Autodesk Inventor part; units mm, degrees
(part 4 of 5)
sketch "Эскиз10" plane through (0, 2, 0) normal (0, 1, 0) x (1, 0, 0)
  circle A0 centre (0, -54) radius 1.6 construction
  line L0 (0, -54) -> (0, -66.038) construction
  line L1 (-10.11, -19.198) -> (10.11, -19.198) construction
  line L2 (10.11, -19.198) -> (10.11, -35.5658) construction
  line L3 (10.11, -58.698) -> (-10.11, -58.698) construction
  line L4 (-10.11, -58.698) -> (-10.11, -55.0209) construction
  circle A1 centre (31.9203, -33.1335) radius 1.6 construction
  circle A2 centre (-31.9203, -33.1335) radius 1.6 construction
  circle A3 centre (21.9203, -33.1335) radius 1.6 construction
  circle A4 centre (-21.9203, -33.1335) radius 1.6 construction
  line L5 (16.2132, -33.1838) -> (7.7166, -24.6871) construction
  arc A5 (8.4003, -21.4111) -> (7.7166, -24.6871) centre (9.1308, -23.2729) ccw construction
  arc A6 (8.4003, -21.4111) -> (21.4111, -8.4003) centre (0, 0) ccw construction
  arc A7 (24.6871, -7.7166) -> (21.4111, -8.4003) centre (23.2729, -9.1308) ccw construction
  line L6 (24.6871, -7.7166) -> (37.8302, -20.8597) construction
  arc A8 (37.8302, -23.6881) -> (37.8302, -20.8597) centre (36.416, -22.2739) ccw construction
  line L7 (37.8302, -23.6881) -> (33.2132, -28.3051) construction
  line L8 (33.2132, -28.3051) -> (21.9203, -28.3051) construction
  arc A9 (21.9203, -28.3051) -> (20.5061, -28.8909) centre (21.9203, -30.3051) ccw construction
  line L9 (20.5061, -28.8909) -> (16.2132, -33.1838) construction
  line L10 (-31.4801, -37.1092) -> (-27.2236, -41.3657) construction
  arc A10 (-27.2236, -44.1942) -> (-27.2236, -41.3657) centre (-28.6378, -42.78) ccw construction
  line L11 (-27.2236, -44.1942) -> (-46.669, -63.6396) construction
  line L12 (-46.669, -63.6396) -> (-63.6396, -46.669) construction
  line L13 (-63.6396, -46.669) -> (-44.1942, -27.2236) construction
  arc A11 (-41.3657, -27.2236) -> (-44.1942, -27.2236) centre (-42.78, -28.6378) ccw construction
  line L14 (-41.3657, -27.2236) -> (-35.896, -32.6933) construction
  arc A12 (-35.896, -32.6933) -> (-31.4801, -37.1092) centre (-31.9203, -33.1335) ccw construction
  circle A13 centre (45.1111, -90.3659) radius 1.6 construction
  circle A14 centre (-45.1111, 90.3659) radius 1.6 construction
  circle A15 centre (-90.3659, 45.1111) radius 1.6 construction
  circle A16 centre (90.3659, -45.1111) radius 1.6 construction
  circle A17 centre (-45.1111, -90.3659) radius 1.6 construction
  circle A18 centre (45.1111, 90.3659) radius 1.6 construction
  circle A19 centre (-90.3659, -45.1111) radius 1.6 construction
  circle A20 centre (90.3659, 45.1111) radius 1.6 construction
  circle A21 centre (101, 0) radius 1.6 construction
  circle A22 centre (-101, 0) radius 1.6 construction
  arc A23 (90.4395, -37.7453) -> (97.9653, -2.6059) centre (0, 0) ccw construction
  arc A24 (87.1795, -38.3892) -> (90.4395, -37.7453) centre (88.5938, -36.975) ccw construction
  line L15 (87.1795, -38.3892) -> (83.085, -34.2947) construction
  arc A25 (83.085, -34.2947) -> (76.014, -34.2947) centre (79.5495, -37.8302) ccw construction
  line L16 (76.014, -34.2947) -> (67.8823, -42.4264) construction
  line L17 (67.8823, -42.4264) -> (47.1257, -21.6698) construction
  arc A26 (47.1257, -21.6698) -> (43.384, -17.9282) centre (43.1335, -21.9203) ccw construction
  line L18 (43.384, -17.9282) -> (26.8701, -1.4142) construction
  arc A27 (26.8701, 1.4142) -> (26.8701, -1.4142) centre (28.2843, 0) ccw construction
  line L19 (26.8701, 1.4142) -> (43.384, 17.9282) construction
  arc A28 (43.384, 17.9282) -> (47.1257, 21.6698) centre (43.1335, 21.9203) ccw construction
  line L20 (47.1257, 21.6698) -> (67.8823, 42.4264) construction
  line L21 (67.8823, 42.4264) -> (76.014, 34.2947) construction
  arc A29 (76.014, 34.2947) -> (83.085, 34.2947) centre (79.5495, 37.8302) ccw construction
  line L22 (83.085, 34.2947) -> (87.1795, 38.3892) construction
  arc A30 (90.4395, 37.7453) -> (87.1795, 38.3892) centre (88.5938, 36.975) ccw construction
  arc A31 (97.9653, 2.6059) -> (90.4395, 37.7453) centre (0, 0) ccw construction
  arc A32 (97.9653, 2.6059) -> (97.9653, -2.6059) centre (101, 0) ccw construction
  arc A33 (3.4868, -52.0398) -> (5.1776, -53.4237) centre (6.1018, -50.5696) ccw projected
  arc A34 (3.4868, -52.0398) -> (-3.4868, -52.0398) centre (0, -54) ccw projected
  arc A35 (-5.1776, -53.4237) -> (-3.4868, -52.0398) centre (-6.1018, -50.5696) ccw projected
  line L23 (-5.1776, -53.4237) -> (-14.5119, -56.4463) projected
  arc A36 (-15.1585, -56.5907) -> (-14.5119, -56.4463) centre (-15.6055, -53.069) ccw projected
  line L24 (-15.1585, -56.5907) -> (-20.596, -57.2809) construction
  line L25 (-20.596, -57.2809) -> (-26.2105, -51.6664) projected
  line L26 (-26.2105, -51.6664) -> (-21.6698, -47.1257) projected
  arc A37 (-21.6698, -47.1257) -> (-17.9282, -43.384) centre (-21.9203, -43.1335) ccw projected
  line L27 (-17.9282, -43.384) -> (-1.4142, -26.8701) projected
  arc A38 (1.4142, -26.8701) -> (-1.4142, -26.8701) centre (0, -28.2843) ccw projected
  line L28 (1.4142, -26.8701) -> (17.9282, -43.384) projected
  arc A39 (17.9282, -43.384) -> (21.6698, -47.1257) centre (21.9203, -43.1335) ccw projected
  line L29 (21.6698, -47.1257) -> (26.2105, -51.6664) projected
  line L30 (26.2105, -51.6664) -> (20.596, -57.2809) projected
  line L31 (20.596, -57.2809) -> (15.1585, -56.5907) projected
  arc A40 (14.5119, -56.4463) -> (15.1585, -56.5907) centre (15.6055, -53.069) ccw construction
  line L32 (14.5119, -56.4463) -> (5.1776, -53.4237) projected
  line L33 (63.6396, 46.669) -> (44.1942, 27.2236) construction
  arc A41 (41.3657, 27.2236) -> (44.1942, 27.2236) centre (42.78, 28.6378) ccw construction
  line L34 (41.3657, 27.2236) -> (27.2236, 41.3657) construction
  arc A42 (27.2236, 44.1942) -> (27.2236, 41.3657) centre (28.6378, 42.78) ccw construction
  line L35 (27.2236, 44.1942) -> (46.669, 63.6396) construction
  line L36 (46.669, 63.6396) -> (63.6396, 46.669) construction
  line L37 (-46.669, 63.6396) -> (-27.2236, 44.1942) construction
  arc A43 (-27.2236, 41.3657) -> (-27.2236, 44.1942) centre (-28.6378, 42.78) ccw construction
  line L38 (-27.2236, 41.3657) -> (-41.3657, 27.2236) construction
  arc A44 (-44.1942, 27.2236) -> (-41.3657, 27.2236) centre (-42.78, 28.6378) ccw construction
  line L39 (-44.1942, 27.2236) -> (-63.6396, 46.669) construction
  line L40 (-63.6396, 46.669) -> (-46.669, 63.6396) construction
  circle A45 centre (-21.9203, 43.1335) radius 1.6 construction
  arc A46 (-24.6871, 7.7166) -> (-21.4111, 8.4003) centre (-23.2729, 9.1308) ccw construction
  line L41 (-24.6871, 7.7166) -> (-37.8302, 20.8597) construction
  arc A47 (-37.8302, 23.6881) -> (-37.8302, 20.8597) centre (-36.416, 22.2739) ccw construction
  line L42 (-37.8302, 23.6881) -> (-23.6881, 37.8302) construction
  arc A48 (-20.8597, 37.8302) -> (-23.6881, 37.8302) centre (-22.2739, 36.416) ccw construction
  line L43 (-20.8597, 37.8302) -> (-7.7166, 24.6871) construction
  arc A49 (-8.4003, 21.4111) -> (-7.7166, 24.6871) centre (-9.1308, 23.2729) ccw construction
  arc A50 (-8.4003, 21.4111) -> (-21.4111, 8.4003) centre (0, 0) ccw construction
  line L44 (37.8302, 20.8597) -> (24.6871, 7.7166) construction
  arc A51 (21.4111, 8.4003) -> (24.6871, 7.7166) centre (23.2729, 9.1308) ccw construction
  arc A52 (21.4111, 8.4003) -> (8.4003, 21.4111) centre (0, 0) ccw construction
  arc A53 (7.7166, 24.6871) -> (8.4003, 21.4111) centre (9.1308, 23.2729) ccw construction
  line L45 (7.7166, 24.6871) -> (20.8597, 37.8302) construction
  arc A54 (23.6881, 37.8302) -> (20.8597, 37.8302) centre (22.2739, 36.416) ccw construction
  line L46 (23.6881, 37.8302) -> (37.8302, 23.6881) construction
  arc A55 (37.8302, 20.8597) -> (37.8302, 23.6881) centre (36.416, 22.2739) ccw construction
  circle A56 centre (21.9203, -43.1335) radius 1.6 construction
  circle A57 centre (-43.1335, -21.9203) radius 1.6 construction
  circle A58 centre (43.1335, 21.9203) radius 1.6 construction
  circle A59 centre (21.9203, 43.1335) radius 1.6 construction
  circle A60 centre (-21.9203, -43.1335) radius 1.6 construction
  circle A61 centre (-43.1335, 21.9203) radius 1.6 construction
  circle A62 centre (0, 0) radius 18 construction
  circle A63 centre (43.1335, -21.9203) radius 1.6 construction
  circle A64 centre (0, 22) radius 1.6 construction
  circle A65 centre (-22, 0) radius 1.6 construction
  circle A66 centre (0, -22) radius 1.6 construction
  circle A67 centre (22, 0) radius 1.6 construction
  circle A68 centre (-37.8302, 79.5495) radius 1.6 construction
  circle A69 centre (-79.5495, 37.8302) radius 1.6 construction
  circle A70 centre (-79.5495, -37.8302) radius 1.6 construction
  circle A71 centre (79.5495, -37.8302) radius 1.6 construction
  circle A72 centre (37.8302, 79.5495) radius 1.6 construction
  circle A73 centre (79.5495, 37.8302) radius 1.6 construction
  circle A74 centre (-20.5578, -60.8546) radius 1.55 construction
  circle A75 centre (20.5578, -60.8546) radius 1.55 construction
  circle A76 centre (37.8302, -79.5495) radius 1.6 construction
  circle A77 centre (-37.8302, -79.5495) radius 1.6 construction
  line L47 (-33.2132, -28.3051) -> (-37.8302, -23.6881) construction
  arc A78 (-37.8302, -20.8597) -> (-37.8302, -23.6881) centre (-36.416, -22.2739) ccw construction
  line L48 (-37.8302, -20.8597) -> (-24.6871, -7.7166) construction
  arc A79 (-21.4111, -8.4003) -> (-24.6871, -7.7166) centre (-23.2729, -9.1308) ccw construction
  arc A80 (-21.4111, -8.4003) -> (-8.4003, -21.4111) centre (0, 0) ccw projected
  arc A81 (-7.7166, -24.6871) -> (-8.4003, -21.4111) centre (-9.1308, -23.2729) ccw projected
  line L49 (-7.7166, -24.6871) -> (-16.2132, -33.1838) projected
  line L50 (-16.2132, -33.1838) -> (-20.5061, -28.8909) construction
  arc A82 (-20.5061, -28.8909) -> (-21.9203, -28.3051) centre (-21.9203, -30.3051) ccw construction
  line L51 (-21.9203, -28.3051) -> (-33.2132, -28.3051) construction
  arc A83 (37.7453, 90.4395) -> (18.0526, 96.3229) centre (0, 0) ccw construction
  arc A84 (38.3892, 87.1795) -> (37.7453, 90.4395) centre (36.975, 88.5938) ccw construction
  line L52 (38.3892, 87.1795) -> (34.2947, 83.085) construction
  arc A85 (34.2947, 83.085) -> (34.2947, 76.014) centre (37.8302, 79.5495) ccw construction
  line L53 (34.2947, 76.014) -> (42.4264, 67.8823) construction
  line L54 (42.4264, 67.8823) -> (21.6698, 47.1257) construction
  arc A86 (21.6698, 47.1257) -> (17.9282, 43.384) centre (21.9203, 43.1335) ccw construction
  line L55 (17.9282, 43.384) -> (1.4142, 26.8701) construction
  arc A87 (-1.4142, 26.8701) -> (1.4142, 26.8701) centre (0, 28.2843) ccw construction
  line L56 (-1.4142, 26.8701) -> (-17.9282, 43.384) construction
  arc A88 (-17.9282, 43.384) -> (-21.6698, 47.1257) centre (-21.9203, 43.1335) ccw construction
  line L57 (-21.6698, 47.1257) -> (-42.4264, 67.8823) construction
  line L58 (-42.4264, 67.8823) -> (-34.2947, 76.014) construction
  arc A89 (-34.2947, 76.014) -> (-34.2947, 83.085) centre (-37.8302, 79.5495) ccw construction
  line L59 (-34.2947, 83.085) -> (-38.3892, 87.1795) construction
  arc A90 (-37.7453, 90.4395) -> (-38.3892, 87.1795) centre (-36.975, 88.5938) ccw construction
  arc A91 (-18.0526, 96.3229) -> (-37.7453, 90.4395) centre (0, 0) ccw construction
  arc A92 (-14.5, 93.3742) -> (-18.0526, 96.3229) centre (-17.5, 93.3742) ccw construction
  line L60 (-14.5, 93.3742) -> (-14.5, 87) construction
  arc A93 (-14.5, 87) -> (-11.5, 84) centre (-11.5, 87) ccw construction
  line L61 (-11.5, 84) -> (11.5, 84) construction
  arc A94 (11.5, 84) -> (14.5, 87) centre (11.5, 87) ccw construction
  line L62 (14.5, 87) -> (14.5, 93.3742) construction
  arc A95 (18.0526, 96.3229) -> (14.5, 93.3742) centre (17.5, 93.3742) ccw construction
  line L63 (-24.3148, -60.6331) -> (-24.842, -61.8893) construction
  arc A96 (-25.4187, -62.8242) -> (-24.842, -61.8893) centre (-28.1154, -60.5155) ccw construction
  line L64 (-25.4187, -62.8242) -> (-34.1909, -73.0707) construction
  arc A97 (-37.1244, -73.1843) -> (-34.1909, -73.0707) centre (-35.7102, -71.7701) ccw construction
  line L65 (-37.1244, -73.1843) -> (-42.4264, -67.8823) construction
  line L66 (-42.4264, -67.8823) -> (-29.746, -55.2019) construction
  line L67 (-29.746, -55.2019) -> (-24.3148, -60.6331) construction
  line L68 (29.746, -55.2019) -> (42.4264, -67.8823) construction
  line L69 (42.4264, -67.8823) -> (37.1244, -73.1843) construction
  arc A98 (34.1909, -73.0707) -> (37.1244, -73.1843) centre (35.7102, -71.7701) ccw construction
  line L70 (34.1909, -73.0707) -> (25.4187, -62.8242) construction
  arc A99 (24.842, -61.8893) -> (25.4187, -62.8242) centre (28.1154, -60.5155) ccw construction
  line L71 (24.842, -61.8893) -> (24.3148, -60.6331) construction
  line L72 (24.3148, -60.6331) -> (29.746, -55.2019) construction
  arc A100 (-90.4395, 37.7453) -> (-97.9653, 2.6059) centre (0, 0) ccw construction
  arc A101 (-87.1795, 38.3892) -> (-90.4395, 37.7453) centre (-88.5938, 36.975) ccw construction
  line L73 (-87.1795, 38.3892) -> (-83.085, 34.2947) construction
  arc A102 (-83.085, 34.2947) -> (-76.014, 34.2947) centre (-79.5495, 37.8302) ccw construction
  line L74 (-76.014, 34.2947) -> (-67.8823, 42.4264) construction
  line L75 (-67.8823, 42.4264) -> (-47.1257, 21.6698) construction
  arc A103 (-47.1257, 21.6698) -> (-43.384, 17.9282) centre (-43.1335, 21.9203) ccw construction
  line L76 (-43.384, 17.9282) -> (-26.8701, 1.4142) construction
  arc A104 (-26.8701, -1.4142) -> (-26.8701, 1.4142) centre (-28.2843, 0) ccw construction
  line L77 (-26.8701, -1.4142) -> (-43.384, -17.9282) construction
  arc A105 (-43.384, -17.9282) -> (-47.1257, -21.6698) centre (-43.1335, -21.9203) ccw construction
  line L78 (-47.1257, -21.6698) -> (-67.8823, -42.4264) construction
  line L79 (-67.8823, -42.4264) -> (-76.014, -34.2947) construction
  arc A106 (-76.014, -34.2947) -> (-83.085, -34.2947) centre (-79.5495, -37.8302) ccw construction
  line L80 (-83.085, -34.2947) -> (-87.1795, -38.3892) construction
  arc A107 (-90.4395, -37.7453) -> (-87.1795, -38.3892) centre (-88.5938, -36.975) ccw construction
  arc A108 (-97.9653, -2.6059) -> (-90.4395, -37.7453) centre (0, 0) ccw construction
  arc A109 (-97.9653, -2.6059) -> (-97.9653, 2.6059) centre (-101, 0) ccw construction
  arc A110 (-93.0503, 48.6481) -> (-93.0503, -48.6481) centre (0, 0) ccw construction
  arc A111 (-93.0503, -48.6481) -> (-88.2704, -49.3795) centre (-90.3917, -47.2582) ccw construction
  line L81 (-88.2704, -49.3795) -> (-85.2064, -46.3155) construction
  arc A112 (-73.8927, -46.3155) -> (-85.2064, -46.3155) centre (-79.5495, -51.9723) ccw construction
  line L82 (-73.8927, -46.3155) -> (-46.3155, -73.8927) construction
  arc A113 (-46.3155, -85.2064) -> (-46.3155, -73.8927) centre (-51.9723, -79.5495) ccw construction
  line L83 (-46.3155, -85.2064) -> (-49.3795, -88.2704) construction
  arc A114 (-49.3795, -88.2704) -> (-48.6481, -93.0503) centre (-47.2582, -90.3917) ccw construction
  arc A115 (-48.6481, -93.0503) -> (-45.42, -94.668) centre (0, 0) ccw construction
  arc A116 (-45.42, -94.668) -> (-43.0355, -94.1655) centre (-44.5548, -92.8648) ccw construction
  line L84 (-43.0355, -94.1655) -> (-18.3802, -65.3664) construction
  arc A117 (-17.477, -64.7643) -> (-18.3802, -65.3664) centre (-16.8609, -66.6671) ccw construction
  line L85 (-17.477, -64.7643) -> (-0.6161, -59.3045) construction
  arc A118 (0.6161, -59.3045) -> (-0.6161, -59.3045) centre (0, -61.2072) ccw construction
  line L86 (0.6161, -59.3045) -> (17.477, -64.7643) construction
  arc A119 (18.3802, -65.3664) -> (17.477, -64.7643) centre (16.8609, -66.6671) ccw construction
  line L87 (18.3802, -65.3664) -> (43.0355, -94.1655) construction
  arc A120 (43.0355, -94.1655) -> (45.42, -94.668) centre (44.5548, -92.8648) ccw construction
  arc A121 (45.42, -94.668) -> (48.6481, -93.0503) centre (0, 0) ccw construction
  arc A122 (48.6481, -93.0503) -> (49.3795, -88.2704) centre (47.2582, -90.3917) ccw construction
  line L88 (49.3795, -88.2704) -> (46.3155, -85.2064) construction
  arc A123 (46.3155, -73.8927) -> (46.3155, -85.2064) centre (51.9723, -79.5495) ccw construction
  line L89 (46.3155, -73.8927) -> (73.8927, -46.3155) construction
  arc A124 (85.2064, -46.3155) -> (73.8927, -46.3155) centre (79.5495, -51.9723) ccw construction
  line L90 (85.2064, -46.3155) -> (88.2704, -49.3795) construction
  arc A125 (88.2704, -49.3795) -> (93.0503, -48.6481) centre (90.3917, -47.2582) ccw construction
  arc A126 (93.0503, -48.6481) -> (93.0503, 48.6481) centre (0, 0) ccw construction
  arc A127 (93.0503, 48.6481) -> (88.2704, 49.3795) centre (90.3917, 47.2582) ccw construction
  line L91 (88.2704, 49.3795) -> (85.2064, 46.3155) construction
  arc A128 (73.8927, 46.3155) -> (85.2064, 46.3155) centre (79.5495, 51.9723) ccw construction
  line L92 (73.8927, 46.3155) -> (46.3155, 73.8927) construction
  arc A129 (46.3155, 85.2064) -> (46.3155, 73.8927) centre (51.9723, 79.5495) ccw construction
  line L93 (46.3155, 85.2064) -> (49.3795, 88.2704) construction
  arc A130 (49.3795, 88.2704) -> (48.6481, 93.0503) centre (47.2582, 90.3917) ccw construction
  arc A131 (48.6481, 93.0503) -> (11.8382, 104.3305) centre (0, 0) ccw construction
  arc A132 (11.8382, 104.3305) -> (8.5, 101.3496) centre (11.5, 101.3496) ccw construction
  line L94 (8.5, 101.3496) -> (8.5, 90.5) construction
  arc A133 (7, 89) -> (8.5, 90.5) centre (7, 90.5) ccw construction
  line L95 (7, 89) -> (-7, 89) construction
  arc A134 (-8.5, 90.5) -> (-7, 89) centre (-7, 90.5) ccw construction
  line L96 (-8.5, 90.5) -> (-8.5, 101.3496) construction
  arc A135 (-8.5, 101.3496) -> (-11.8382, 104.3305) centre (-11.5, 101.3496) ccw construction
  arc A136 (-11.8382, 104.3305) -> (-48.6481, 93.0503) centre (0, 0) ccw construction
  arc A137 (-48.6481, 93.0503) -> (-49.3795, 88.2704) centre (-47.2582, 90.3917) ccw construction
  line L97 (-49.3795, 88.2704) -> (-46.3155, 85.2064) construction
  arc A138 (-46.3155, 73.8927) -> (-46.3155, 85.2064) centre (-51.9723, 79.5495) ccw construction
  line L98 (-46.3155, 73.8927) -> (-73.8927, 46.3155) construction
  arc A139 (-85.2064, 46.3155) -> (-73.8927, 46.3155) centre (-79.5495, 51.9723) ccw construction
  line L99 (-85.2064, 46.3155) -> (-88.2704, 49.3795) construction
  arc A140 (-88.2704, 49.3795) -> (-93.0503, 48.6481) centre (-90.3917, 47.2582) ccw construction
  circle A141 centre (0, -54) radius 1.6 construction
  line L100 (35.896, -32.6933) -> (41.3657, -27.2236) construction
  arc A142 (44.1942, -27.2236) -> (41.3657, -27.2236) centre (42.78, -28.6378) ccw construction
  line L101 (44.1942, -27.2236) -> (63.6396, -46.669) construction
  line L102 (63.6396, -46.669) -> (46.669, -63.6396) construction
  line L103 (46.669, -63.6396) -> (27.2236, -44.1942) construction
  arc A143 (27.2236, -41.3657) -> (27.2236, -44.1942) centre (28.6378, -42.78) ccw construction
  line L104 (27.2236, -41.3657) -> (31.4801, -37.1092) construction
  arc A144 (31.4801, -37.1092) -> (35.896, -32.6933) centre (31.9203, -33.1335) ccw construction
  line L105 (0, -22) -> (0, -54) construction
  circle A145 centre (7.01, -46.7128) radius 1.75
  circle A146 centre (-7.01, -24.698) radius 1.75
  line L106 (-16.2132, -33.1838) -> (-7.7166, -24.6871) projected
  line L107 (-11.01, -27.9806) -> (-11.01, -20.1936)
  arc A147 (-21.4111, -8.4003) -> (-8.4003, -21.4111) centre (0, 0) ccw projected
  line L108 (10.11, -35.5658) -> (10.11, -55.0209)
  line L109 (10.11, -55.0209) -> (10.11, -58.698) construction
  line L110 (-10.11, -55.0209) -> (-10.11, -35.5658)
  line L111 (-10.11, -35.5658) -> (-10.11, -19.198) construction
  line L112 (-17.9282, -43.384) -> (-17.9282, -56.9423)
  line L113 (-15.1585, -56.5907) -> (-20.596, -57.2809) projected
  line L114 (17.9282, -43.384) -> (17.9282, -56.9423)
  line L115 (-8.1, -30.338) -> (8.1, -30.338) construction
  line L116 (8.1, -30.338) -> (8.1, -60.538) construction
  line L117 (8.1, -60.538) -> (-8.1, -60.538) construction
  line L118 (-8.1, -60.538) -> (-8.1, -30.338) construction
  circle A148 centre (-3.6, -36.138) radius 1.5
  circle A149 centre (5, -40.8369) radius 1.5
  circle A150 centre (3.6, -51.4954) radius 1.5
  circle A151 centre (-5, -53.3813) radius 1.5
  point P0 (-8.553, -25.5236)
  point P1 (-7.1564, -22.9541)
  dimension "d26" = 360
  dimension "d141" = 12.038
  dimension "d142" = 7.34
  dimension "d143" = 3.5
  dimension "d145" = 39.5
  dimension "d147" = 3.5
  dimension "d148" = 3.1
  dimension "d149" = 5.5
  dimension "d150" = 26.1
  dimension "d151" = 4
  dimension "d152" = 3.1
  dimension "d153" = 20.22
  dimension "d171" = 5.5
  dimension "d172" = 30.2
  dimension "d173" = 16.2
  dimension "d174" = 3
  dimension "d175" = 4.5
  dimension "d176" = 3
  dimension "d177" = 3.1
  dimension "d178" = 5.8
  dimension "d179" = 9.8
  dimension "d180" = 3
  dimension "d181" = 4.5
  dimension "d182" = 10.75
  dimension "d183" = 3
  dimension "d184" = 3.1
  dimension "d185" = 16.0424
  dimension "d186" = 17.3
  constraints: 34 end point, 12 parallel, 6 centre point, 6 point on line, 4 perpendicular, 4 vertical, 2 horizontal, 1 point on circle, 1 symmetric about line, 2 other
  measures "d141" distance of L0.start L0.end
  measures "d142" distance from line of L3 L0.end
  measures "d143" diameter of A145
  measures "d145" distance between parallel lines of L3 L1
  measures "d147" diameter of A146
  measures "d148" distance from line of L4 A146.centre
  measures "d149" distance from line of L1 A146.centre
  measures "d150" distance of A145.centre A146.centre
  measures "d151" distance from line of A146.centre L107
  measures "d152" distance from line of L108 A145.centre
  measures "d153" distance between parallel lines of L111 L2
  measures "d171" distance from line of L0.end L117
  measures "d172" distance between parallel lines of L115 L117
  measures "d173" distance between parallel lines of L118 L116
  measures "d174" diameter of A148
  measures "d175" distance from line of L118 A148.centre
  measures "d176" diameter of A149
  measures "d177" distance from line of L116 A149.centre
  measures "d178" distance from line of L115 A148.centre
  measures "d179" distance of A148.centre A149.centre
  measures "d180" diameter of A150
  measures "d181" distance from line of L116 A150.centre
  measures "d182" distance of A150.centre A149.centre
  measures "d183" diameter of A151
  measures "d184" distance from line of L118 A151.centre
  measures "d185" distance of A151.centre A149.centre
  measures "d186" distance of A151.centre A148.centre
extrude "Выдавливание13" add sketch "Эскиз10" against normal up to surface (2 mm away) contours A34 A150 A33 | A150 A34 A35 A151 L23 L110 L27 A38 L28 L108 L32 A33 | A35 L23 A151 | L112 L113 L25 L26 A37 | A39 L29 L30 L31 L114 | A80 A81 A146 L49 L107 | A148 | A149 picked at (3.8604, -51.4659) picked at (-5.0634, -52.8492)
extrude "Выдавливание14" cut sketch "Эскиз10" along normal mid plane 33.2 contours A146 L49 A81 picked at (-7.051, -25.0464)
fillet "Сопряжение1" radius 2 2 edges at (-10.11, 1, 35.5658) (10.11, 1, 35.5658)
chamfer "Фаска1" distance 4 angle 45 2 edges at (-16.2132, 1, 33.1838) (16.2132, 1, 33.1838)
sketch "Эскиз11" plane through (0, 2, 0) normal (0, 1, 0) x (1, 0, 0)
  line L0 (35.896, -32.6933) -> (41.3657, -27.2236) projected
  arc A0 (44.1942, -27.2236) -> (41.3657, -27.2236) centre (42.78, -28.6378) ccw projected
  line L1 (44.1942, -27.2236) -> (63.6396, -46.669) projected
  line L2 (63.6396, -46.669) -> (46.669, -63.6396) projected
  line L3 (46.669, -63.6396) -> (27.2236, -44.1942) projected
  arc A1 (27.2236, -41.3657) -> (27.2236, -44.1942) centre (28.6378, -42.78) ccw projected
  line L4 (27.2236, -41.3657) -> (31.4801, -37.1092) projected
  arc A2 (31.4801, -37.1092) -> (35.896, -32.6933) centre (31.9203, -33.1335) ccw projected
  circle A3 centre (0, -54) radius 1.6 projected
  arc A4 (-93.0503, 48.6481) -> (-93.0503, -48.6481) centre (0, 0) ccw projected
  arc A5 (-93.0503, -48.6481) -> (-88.2704, -49.3795) centre (-90.3917, -47.2582) ccw projected
  line L5 (-88.2704, -49.3795) -> (-85.2064, -46.3155) projected
  arc A6 (-73.8927, -46.3155) -> (-85.2064, -46.3155) centre (-79.5495, -51.9723) ccw projected
  line L6 (-73.8927, -46.3155) -> (-46.3155, -73.8927) projected
  arc A7 (-46.3155, -85.2064) -> (-46.3155, -73.8927) centre (-51.9723, -79.5495) ccw projected
  line L7 (-46.3155, -85.2064) -> (-49.3795, -88.2704) projected
  arc A8 (-49.3795, -88.2704) -> (-48.6481, -93.0503) centre (-47.2582, -90.3917) ccw projected
  arc A9 (-48.6481, -93.0503) -> (-45.42, -94.668) centre (0, 0) ccw projected
  arc A10 (-45.42, -94.668) -> (-43.0355, -94.1655) centre (-44.5548, -92.8648) ccw projected
  line L8 (-43.0355, -94.1655) -> (-18.3802, -65.3664) projected
  arc A11 (-17.477, -64.7643) -> (-18.3802, -65.3664) centre (-16.8609, -66.6671) ccw projected
  line L9 (-17.477, -64.7643) -> (-0.6161, -59.3045) projected
  arc A12 (0.6161, -59.3045) -> (-0.6161, -59.3045) centre (0, -61.2072) ccw projected
  line L10 (0.6161, -59.3045) -> (17.477, -64.7643) projected
  arc A13 (18.3802, -65.3664) -> (17.477, -64.7643) centre (16.8609, -66.6671) ccw projected
  line L11 (18.3802, -65.3664) -> (43.0355, -94.1655) projected
  arc A14 (43.0355, -94.1655) -> (45.42, -94.668) centre (44.5548, -92.8648) ccw projected
  arc A15 (45.42, -94.668) -> (48.6481, -93.0503) centre (0, 0) ccw projected
  arc A16 (48.6481, -93.0503) -> (49.3795, -88.2704) centre (47.2582, -90.3917) ccw projected
  line L12 (49.3795, -88.2704) -> (46.3155, -85.2064) projected
  arc A17 (46.3155, -73.8927) -> (46.3155, -85.2064) centre (51.9723, -79.5495) ccw projected
  line L13 (46.3155, -73.8927) -> (73.8927, -46.3155) projected
  arc A18 (85.2064, -46.3155) -> (73.8927, -46.3155) centre (79.5495, -51.9723) ccw projected
  line L14 (85.2064, -46.3155) -> (88.2704, -49.3795) projected
  arc A19 (88.2704, -49.3795) -> (93.0503, -48.6481) centre (90.3917, -47.2582) ccw projected
  arc A20 (93.0503, -48.6481) -> (93.0503, 48.6481) centre (0, 0) ccw projected
  arc A21 (93.0503, 48.6481) -> (88.2704, 49.3795) centre (90.3917, 47.2582) ccw projected
  line L15 (88.2704, 49.3795) -> (85.2064, 46.3155) projected
  arc A22 (73.8927, 46.3155) -> (85.2064, 46.3155) centre (79.5495, 51.9723) ccw projected
  line L16 (73.8927, 46.3155) -> (46.3155, 73.8927) projected
  arc A23 (46.3155, 85.2064) -> (46.3155, 73.8927) centre (51.9723, 79.5495) ccw projected
  line L17 (46.3155, 85.2064) -> (49.3795, 88.2704) projected
  arc A24 (49.3795, 88.2704) -> (48.6481, 93.0503) centre (47.2582, 90.3917) ccw projected
  arc A25 (48.6481, 93.0503) -> (11.8382, 104.3305) centre (0, 0) ccw projected
  arc A26 (11.8382, 104.3305) -> (8.5, 101.3496) centre (11.5, 101.3496) ccw projected
  line L18 (8.5, 101.3496) -> (8.5, 90.5) projected
  arc A27 (7, 89) -> (8.5, 90.5) centre (7, 90.5) ccw projected
  line L19 (7, 89) -> (-7, 89) projected
  arc A28 (-8.5, 90.5) -> (-7, 89) centre (-7, 90.5) ccw projected
  line L20 (-8.5, 90.5) -> (-8.5, 101.3496) projected
  arc A29 (-8.5, 101.3496) -> (-11.8382, 104.3305) centre (-11.5, 101.3496) ccw projected
  arc A30 (-11.8382, 104.3305) -> (-48.6481, 93.0503) centre (0, 0) ccw projected
  arc A31 (-48.6481, 93.0503) -> (-49.3795, 88.2704) centre (-47.2582, 90.3917) ccw projected
  line L21 (-49.3795, 88.2704) -> (-46.3155, 85.2064) projected
  arc A32 (-46.3155, 73.8927) -> (-46.3155, 85.2064) centre (-51.9723, 79.5495) ccw projected
  line L22 (-46.3155, 73.8927) -> (-73.8927, 46.3155) projected
  arc A33 (-85.2064, 46.3155) -> (-73.8927, 46.3155) centre (-79.5495, 51.9723) ccw projected
  line L23 (-85.2064, 46.3155) -> (-88.2704, 49.3795) projected
  arc A34 (-88.2704, 49.3795) -> (-93.0503, 48.6481) centre (-90.3917, 47.2582) ccw projected
  arc A35 (-90.4395, 37.7453) -> (-97.9653, 2.6059) centre (0, 0) ccw projected
  arc A36 (-87.1795, 38.3892) -> (-90.4395, 37.7453) centre (-88.5938, 36.975) ccw projected
  line L24 (-87.1795, 38.3892) -> (-83.085, 34.2947) projected
  arc A37 (-83.085, 34.2947) -> (-76.014, 34.2947) centre (-79.5495, 37.8302) ccw projected
  line L25 (-76.014, 34.2947) -> (-67.8823, 42.4264) projected
  line L26 (-67.8823, 42.4264) -> (-47.1257, 21.6698) projected
  arc A38 (-47.1257, 21.6698) -> (-43.384, 17.9282) centre (-43.1335, 21.9203) ccw projected
  line L27 (-43.384, 17.9282) -> (-26.8701, 1.4142) projected
  arc A39 (-26.8701, -1.4142) -> (-26.8701, 1.4142) centre (-28.2843, 0) ccw projected
  line L28 (-26.8701, -1.4142) -> (-43.384, -17.9282) projected
  arc A40 (-43.384, -17.9282) -> (-47.1257, -21.6698) centre (-43.1335, -21.9203) ccw projected
  line L29 (-47.1257, -21.6698) -> (-67.8823, -42.4264) projected
  line L30 (-67.8823, -42.4264) -> (-76.014, -34.2947) projected
  arc A41 (-76.014, -34.2947) -> (-83.085, -34.2947) centre (-79.5495, -37.8302) ccw projected
  line L31 (-83.085, -34.2947) -> (-87.1795, -38.3892) projected
  arc A42 (-90.4395, -37.7453) -> (-87.1795, -38.3892) centre (-88.5938, -36.975) ccw projected
  arc A43 (-97.9653, -2.6059) -> (-90.4395, -37.7453) centre (0, 0) ccw projected
  arc A44 (-97.9653, -2.6059) -> (-97.9653, 2.6059) centre (-101, 0) ccw projected
  line L32 (29.746, -55.2019) -> (42.4264, -67.8823) projected
  line L33 (42.4264, -67.8823) -> (37.1244, -73.1843) projected
  arc A45 (34.1909, -73.0707) -> (37.1244, -73.1843) centre (35.7102, -71.7701) ccw projected
  line L34 (34.1909, -73.0707) -> (25.4187, -62.8242) projected
  arc A46 (24.842, -61.8893) -> (25.4187, -62.8242) centre (28.1154, -60.5155) ccw projected
  line L35 (24.842, -61.8893) -> (24.3148, -60.6331) projected
  line L36 (24.3148, -60.6331) -> (29.746, -55.2019) projected
  line L37 (-24.3148, -60.6331) -> (-24.842, -61.8893) projected
  arc A47 (-25.4187, -62.8242) -> (-24.842, -61.8893) centre (-28.1154, -60.5155) ccw projected
  line L38 (-25.4187, -62.8242) -> (-34.1909, -73.0707) projected
  arc A48 (-37.1244, -73.1843) -> (-34.1909, -73.0707) centre (-35.7102, -71.7701) ccw projected
  line L39 (-37.1244, -73.1843) -> (-42.4264, -67.8823) projected
  line L40 (-42.4264, -67.8823) -> (-29.746, -55.2019) projected
  line L41 (-29.746, -55.2019) -> (-24.3148, -60.6331) projected
  arc A49 (37.7453, 90.4395) -> (18.0526, 96.3229) centre (0, 0) ccw projected
  arc A50 (38.3892, 87.1795) -> (37.7453, 90.4395) centre (36.975, 88.5938) ccw projected
  line L42 (38.3892, 87.1795) -> (34.2947, 83.085) projected
  arc A51 (34.2947, 83.085) -> (34.2947, 76.014) centre (37.8302, 79.5495) ccw projected
  line L43 (34.2947, 76.014) -> (42.4264, 67.8823) projected
  line L44 (42.4264, 67.8823) -> (21.6698, 47.1257) projected
  arc A52 (21.6698, 47.1257) -> (17.9282, 43.384) centre (21.9203, 43.1335) ccw projected
  line L45 (17.9282, 43.384) -> (1.4142, 26.8701) projected
  arc A53 (-1.4142, 26.8701) -> (1.4142, 26.8701) centre (0, 28.2843) ccw projected
  line L46 (-1.4142, 26.8701) -> (-17.9282, 43.384) projected
  arc A54 (-17.9282, 43.384) -> (-21.6698, 47.1257) centre (-21.9203, 43.1335) ccw projected
  line L47 (-21.6698, 47.1257) -> (-42.4264, 67.8823) projected
  line L48 (-42.4264, 67.8823) -> (-34.2947, 76.014) projected
  arc A55 (-34.2947, 76.014) -> (-34.2947, 83.085) centre (-37.8302, 79.5495) ccw projected
  line L49 (-34.2947, 83.085) -> (-38.3892, 87.1795) projected
  arc A56 (-37.7453, 90.4395) -> (-38.3892, 87.1795) centre (-36.975, 88.5938) ccw projected
  arc A57 (-18.0526, 96.3229) -> (-37.7453, 90.4395) centre (0, 0) ccw projected
  arc A58 (-14.5, 93.3742) -> (-18.0526, 96.3229) centre (-17.5, 93.3742) ccw projected
  line L50 (-14.5, 93.3742) -> (-14.5, 87) projected
  arc A59 (-14.5, 87) -> (-11.5, 84) centre (-11.5, 87) ccw projected
  line L51 (-11.5, 84) -> (11.5, 84) projected
  arc A60 (11.5, 84) -> (14.5, 87) centre (11.5, 87) ccw projected
  line L52 (14.5, 87) -> (14.5, 93.3742) projected
  arc A61 (18.0526, 96.3229) -> (14.5, 93.3742) centre (17.5, 93.3742) ccw projected
  circle A62 centre (-7.01, -24.698) radius 1.75 projected
  circle A63 centre (-37.8302, -79.5495) radius 1.6 projected
  circle A64 centre (37.8302, -79.5495) radius 1.6 projected
  circle A65 centre (20.5578, -60.8546) radius 1.55 projected
  circle A66 centre (-20.5578, -60.8546) radius 1.55 projected
  circle A67 centre (79.5495, 37.8302) radius 1.6 projected
  circle A68 centre (37.8302, 79.5495) radius 1.6 projected
  circle A69 centre (79.5495, -37.8302) radius 1.6 projected
  circle A70 centre (-79.5495, -37.8302) radius 1.6 projected
  circle A71 centre (-79.5495, 37.8302) radius 1.6 projected
  circle A72 centre (-37.8302, 79.5495) radius 1.6 projected
  circle A73 centre (22, 0) radius 1.6 projected
  circle A74 centre (0, -22) radius 1.6 projected
  circle A75 centre (-22, 0) radius 1.6 projected
  circle A76 centre (0, 22) radius 1.6 projected
  circle A77 centre (43.1335, -21.9203) radius 1.6 projected
  circle A78 centre (0, 0) radius 18 projected
  circle A79 centre (-43.1335, 21.9203) radius 1.6 projected
  circle A80 centre (-21.9203, -43.1335) radius 1.6 projected
  circle A81 centre (21.9203, 43.1335) radius 1.6 projected
  circle A82 centre (43.1335, 21.9203) radius 1.6 projected
  circle A83 centre (-43.1335, -21.9203) radius 1.6 projected
  circle A84 centre (21.9203, -43.1335) radius 1.6 projected
  line L53 (37.8302, 20.8597) -> (24.6871, 7.7166) projected
  arc A85 (21.4111, 8.4003) -> (24.6871, 7.7166) centre (23.2729, 9.1308) ccw projected
  arc A86 (21.4111, 8.4003) -> (8.4003, 21.4111) centre (0, 0) ccw projected
  arc A87 (7.7166, 24.6871) -> (8.4003, 21.4111) centre (9.1308, 23.2729) ccw projected
  line L54 (7.7166, 24.6871) -> (20.8597, 37.8302) projected
  arc A88 (23.6881, 37.8302) -> (20.8597, 37.8302) centre (22.2739, 36.416) ccw projected
  line L55 (23.6881, 37.8302) -> (37.8302, 23.6881) projected
  arc A89 (37.8302, 20.8597) -> (37.8302, 23.6881) centre (36.416, 22.2739) ccw projected
  arc A90 (-24.6871, 7.7166) -> (-21.4111, 8.4003) centre (-23.2729, 9.1308) ccw projected
  line L56 (-24.6871, 7.7166) -> (-37.8302, 20.8597) projected
  arc A91 (-37.8302, 23.6881) -> (-37.8302, 20.8597) centre (-36.416, 22.2739) ccw projected
  line L57 (-37.8302, 23.6881) -> (-23.6881, 37.8302) projected
  arc A92 (-20.8597, 37.8302) -> (-23.6881, 37.8302) centre (-22.2739, 36.416) ccw projected
  line L58 (-20.8597, 37.8302) -> (-7.7166, 24.6871) projected
  arc A93 (-8.4003, 21.4111) -> (-7.7166, 24.6871) centre (-9.1308, 23.2729) ccw projected
  arc A94 (-8.4003, 21.4111) -> (-21.4111, 8.4003) centre (0, 0) ccw projected
  circle A95 centre (-21.9203, 43.1335) radius 1.6 projected
  line L59 (-46.669, 63.6396) -> (-27.2236, 44.1942) projected
  arc A96 (-27.2236, 41.3657) -> (-27.2236, 44.1942) centre (-28.6378, 42.78) ccw projected
  line L60 (-27.2236, 41.3657) -> (-41.3657, 27.2236) projected
  arc A97 (-44.1942, 27.2236) -> (-41.3657, 27.2236) centre (-42.78, 28.6378) ccw projected
  line L61 (-44.1942, 27.2236) -> (-63.6396, 46.669) projected
  line L62 (-63.6396, 46.669) -> (-46.669, 63.6396) projected
  line L63 (63.6396, 46.669) -> (44.1942, 27.2236) projected
  arc A98 (41.3657, 27.2236) -> (44.1942, 27.2236) centre (42.78, 28.6378) ccw projected
  line L64 (41.3657, 27.2236) -> (27.2236, 41.3657) projected
  arc A99 (27.2236, 44.1942) -> (27.2236, 41.3657) centre (28.6378, 42.78) ccw projected
  line L65 (27.2236, 44.1942) -> (46.669, 63.6396) projected
  line L66 (46.669, 63.6396) -> (63.6396, 46.669) projected
  line L67 (10.11, -55.0209) -> (10.11, -40.3943) projected
  arc A100 (13.5242, -38.9801) -> (10.11, -40.3943) centre (12.11, -40.3943) ccw projected
  line L68 (13.5242, -38.9801) -> (17.9282, -43.384) projected
  line L69 (17.9282, -56.9423) -> (15.1585, -56.5907) projected
  arc A101 (14.5119, -56.4463) -> (15.1585, -56.5907) centre (15.6055, -53.069) ccw projected
  line L70 (14.5119, -56.4463) -> (10.11, -55.0209) projected
  arc A102 (90.4395, -37.7453) -> (97.9653, -2.6059) centre (0, 0) ccw projected
  arc A103 (87.1795, -38.3892) -> (90.4395, -37.7453) centre (88.5938, -36.975) ccw projected
  line L71 (87.1795, -38.3892) -> (83.085, -34.2947) projected
  arc A104 (83.085, -34.2947) -> (76.014, -34.2947) centre (79.5495, -37.8302) ccw projected
  line L72 (76.014, -34.2947) -> (67.8823, -42.4264) projected
  line L73 (67.8823, -42.4264) -> (47.1257, -21.6698) projected
  arc A105 (47.1257, -21.6698) -> (43.384, -17.9282) centre (43.1335, -21.9203) ccw projected
  line L74 (43.384, -17.9282) -> (26.8701, -1.4142) projected
  arc A106 (26.8701, 1.4142) -> (26.8701, -1.4142) centre (28.2843, 0) ccw projected
  line L75 (26.8701, 1.4142) -> (43.384, 17.9282) projected
  arc A107 (43.384, 17.9282) -> (47.1257, 21.6698) centre (43.1335, 21.9203) ccw projected
  line L76 (47.1257, 21.6698) -> (67.8823, 42.4264) projected
  line L77 (67.8823, 42.4264) -> (76.014, 34.2947) projected
  arc A108 (76.014, 34.2947) -> (83.085, 34.2947) centre (79.5495, 37.8302) ccw projected
  line L78 (83.085, 34.2947) -> (87.1795, 38.3892) projected
  arc A109 (90.4395, 37.7453) -> (87.1795, 38.3892) centre (88.5938, 36.975) ccw projected
  arc A110 (97.9653, 2.6059) -> (90.4395, 37.7453) centre (0, 0) ccw projected
  arc A111 (97.9653, 2.6059) -> (97.9653, -2.6059) centre (101, 0) ccw projected
  circle A112 centre (-101, 0) radius 1.6 projected
  circle A113 centre (101, 0) radius 1.6 projected
  circle A114 centre (90.3659, 45.1111) radius 1.6 projected
  circle A115 centre (-90.3659, -45.1111) radius 1.6 projected
  circle A116 centre (45.1111, 90.3659) radius 1.6 projected
  circle A117 centre (-45.1111, -90.3659) radius 1.6 projected
  circle A118 centre (90.3659, -45.1111) radius 1.6 projected
  circle A119 centre (-90.3659, 45.1111) radius 1.6 projected
  circle A120 centre (-45.1111, 90.3659) radius 1.6 projected
  circle A121 centre (45.1111, -90.3659) radius 1.6 projected
  line L79 (-31.4801, -37.1092) -> (-27.2236, -41.3657) projected
  arc A122 (-27.2236, -44.1942) -> (-27.2236, -41.3657) centre (-28.6378, -42.78) ccw projected
  line L80 (-27.2236, -44.1942) -> (-46.669, -63.6396) projected
  line L81 (-46.669, -63.6396) -> (-63.6396, -46.669) projected
  line L82 (-63.6396, -46.669) -> (-44.1942, -27.2236) projected
  arc A123 (-41.3657, -27.2236) -> (-44.1942, -27.2236) centre (-42.78, -28.6378) ccw projected
  line L83 (-41.3657, -27.2236) -> (-35.896, -32.6933) projected
  arc A124 (-35.896, -32.6933) -> (-31.4801, -37.1092) centre (-31.9203, -33.1335) ccw projected
  line L84 (13.3848, -30.3553) -> (7.7166, -24.6871) projected
  arc A125 (8.4003, -21.4111) -> (7.7166, -24.6871) centre (9.1308, -23.2729) ccw projected
  arc A126 (8.4003, -21.4111) -> (21.4111, -8.4003) centre (0, 0) ccw projected
  arc A127 (24.6871, -7.7166) -> (21.4111, -8.4003) centre (23.2729, -9.1308) ccw projected
  line L85 (24.6871, -7.7166) -> (37.8302, -20.8597) projected
  arc A128 (37.8302, -23.6881) -> (37.8302, -20.8597) centre (36.416, -22.2739) ccw projected
  line L86 (37.8302, -23.6881) -> (33.2132, -28.3051) projected
  line L87 (33.2132, -28.3051) -> (21.9203, -28.3051) projected
  arc A129 (21.9203, -28.3051) -> (20.5061, -28.8909) centre (21.9203, -30.3051) ccw projected
  line L88 (20.5061, -28.8909) -> (19.0416, -30.3553) projected
  line L89 (13.3848, -30.3553) -> (19.0416, -30.3553) projected
  circle A130 centre (-21.9203, -33.1335) radius 1.6 projected
  circle A131 centre (21.9203, -33.1335) radius 1.6 projected
  circle A132 centre (-31.9203, -33.1335) radius 1.6 projected
  circle A133 centre (31.9203, -33.1335) radius 1.6 projected
  circle A134 centre (7.01, -46.7128) radius 1.75 projected
  line L90 (-10.11, -55.0209) -> (-14.5119, -56.4463) projected
  arc A135 (-15.1585, -56.5907) -> (-14.5119, -56.4463) centre (-15.6055, -53.069) ccw projected
  line L91 (-15.1585, -56.5907) -> (-17.9282, -56.9423) projected
  line L92 (-17.9282, -43.384) -> (-13.5242, -38.9801) projected
  arc A136 (-10.11, -40.3943) -> (-13.5242, -38.9801) centre (-12.11, -40.3943) ccw projected
  line L93 (-10.11, -40.3943) -> (-10.11, -55.0209) projected
  line L94 (-11.01, -27.9806) -> (-13.3848, -30.3553) projected
  line L95 (-19.0416, -30.3553) -> (-13.3848, -30.3553) projected
  line L96 (-19.0416, -30.3553) -> (-20.5061, -28.8909) projected
  arc A137 (-20.5061, -28.8909) -> (-21.9203, -28.3051) centre (-21.9203, -30.3051) ccw projected
  line L97 (-21.9203, -28.3051) -> (-33.2132, -28.3051) projected
  line L98 (-33.2132, -28.3051) -> (-37.8302, -23.6881) projected
  arc A138 (-37.8302, -20.8597) -> (-37.8302, -23.6881) centre (-36.416, -22.2739) ccw projected
  line L99 (-37.8302, -20.8597) -> (-24.6871, -7.7166) projected
  arc A139 (-21.4111, -8.4003) -> (-24.6871, -7.7166) centre (-23.2729, -9.1308) ccw projected
  arc A140 (-21.4111, -8.4003) -> (-11.01, -20.1936) centre (0, 0) ccw projected
  line L100 (-11.01, -20.1936) -> (-11.01, -27.9806) projected
  line L101 (-17.9282, -56.9423) -> (-17.9282, -43.384) projected
  line L102 (17.9282, -43.384) -> (17.9282, -56.9423) projected